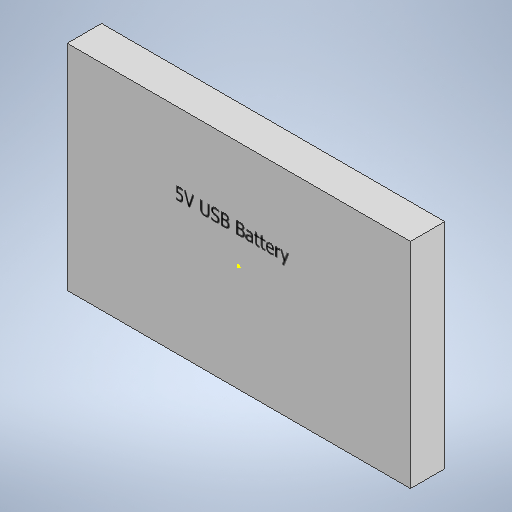
# Autodesk Inventor part: USB-Battery
Saved by Autodesk Inventor 2025.3 (Build 293356000, 356)
## iProperties
Created: 2025-06-02
Part Number: USB-Battery
Material: 一般
Document SubType Name: Modeling
Designer: yamashita1
Density: 1 g/cm^3
Appearance: 既定
Author: yamashita1
Autodesk Inventor part; units mm, degrees
ref_plane "YZ Plane" through (0, 0, 0) normal (1, 0, 0) x (0, 1, 0)
ref_plane "XZ Plane" through (0, 0, 0) normal (0, 1, 0) x (-1, 0, 0)
ref_plane "XY Plane" through (0, 0, 0) normal (0, 0, 1) x (1, 0, 0)
sketch "スケッチ1" plane through (0, 0, 0) normal (0, 0, 1) x (1, 0, 0)
  line L0 (-42.5, 26.5) -> (42.5, 26.5)
  line L1 (42.5, 26.5) -> (42.5, -26.5)
  line L2 (42.5, -26.5) -> (-42.5, -26.5)
  line L3 (-42.5, -26.5) -> (-42.5, 26.5)
  point P0 (0, 0)
  point P1 (-42.5, 0)
  point P2 (0, 26.5)
  dimension "d0" = 85
  dimension "d1" = 53
  constraints: 8 end point, 2 midpoint, 2 parallel, 1 horizontal, 1 horizontal alignment, 1 perpendicular, 1 vertical alignment
  measures "d0" distance of L1.end L2.end
  measures "d1" distance of L0.end L1.end
extrude "押し出し1" add sketch "スケッチ1" along normal blind 8.5
sketch "スケッチ2" plane through (0, 0, 8.5) normal (0, 0, 1) x (1, 0, 0)
  line L0 (-15.8545, 9.585) -> (12.3877, 9.585) construction
  line L1 (12.3877, 9.585) -> (12.3877, 5.6404) construction
  line L2 (12.3877, 5.6404) -> (-15.8545, 5.6404) construction
  line L3 (-15.8545, 5.6404) -> (-15.8545, 9.585) construction
  point P0 (0, 0)
  constraints: 2 other
